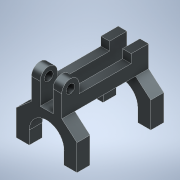
# Autodesk Inventor part: TransferFork
Saved by Autodesk Inventor 2022.2 (Build 262287030, 287C)
## iProperties
Created: 2023-03-20
Part Number: TransferFork
Material: Iron, Cast
Document SubType Name: Modeling
Designer: jak27277
Density: 7.15 g/cm^3
Appearance: Iron Gray
Author: jak27277
Autodesk Inventor part; units mm, degrees
ref_plane "YZ Plane" through (0, 0, 0) normal (1, 0, 0) x (0, 1, 0)
ref_plane "XZ Plane" through (0, 0, 0) normal (0, 1, 0) x (-1, 0, 0)
ref_plane "XY Plane" through (0, 0, 0) normal (0, 0, 1) x (1, 0, 0)
sketch "Sketch1" plane through (0, 0, 0) normal (0, 0, 1) x (1, 0, 0)
  arc A0 (25.4, 0) -> (-25.4, 0) centre (0, 0) ccw
  line L0 (-25.4, 0) -> (-25.4, -19.05)
  line L1 (-25.4, -19.05) -> (-44.45, -19.05)
  line L2 (-44.45, -19.05) -> (-44.45, 19.05)
  line L3 (-44.45, 19.05) -> (-22.225, 38.1)
  line L4 (-22.225, 38.1) -> (-22.225, 69.85)
  line L5 (-22.225, 69.85) -> (-9.525, 69.85)
  line L6 (-9.525, 69.85) -> (-9.525, 38.1)
  line L7 (-9.525, 38.1) -> (0, 38.1)
  line L8 (0, 38.1) -> (0, -30.0357)
  line L9 (25.4, 0) -> (25.4, -19.05)
  line L10 (25.4, -19.05) -> (44.45, -19.05)
  line L11 (44.45, -19.05) -> (44.45, 19.05)
  line L12 (44.45, 19.05) -> (22.225, 38.1)
  line L13 (22.225, 38.1) -> (22.225, 69.85)
  line L14 (9.525, 69.85) -> (9.525, 38.1)
  line L15 (22.225, 69.85) -> (9.525, 69.85)
  line L16 (9.525, 38.1) -> (0, 38.1)
  dimension "d0" = 88.9
  dimension "d1" = 19.05
  dimension "d2" = 38.1
  dimension "d3" = 31.75
  dimension "d4" = 19.05
  dimension "d5" = 25.4
  dimension "d6" = 88.9
  dimension "d7" = 19.05
  dimension "d8" = 44.45
  constraints: 34 end point, 7 symmetric about line, 6 perpendicular, 2 parallel, 2 point on circle, 2 tangent, 2 vertical, 1 centre point, 1 coincident
  measures "d0" distance between parallel lines of L11 L2
  measures "d1" distance of L0.start L0.end
  measures "d2" distance of L11.start L11.end
  measures "d3" distance of L13.start L13.end
  measures "d4" distance of L0.end L1.end
  measures "d5" radius of A0
  measures "d6" distance between parallel lines of L10 L15
  measures "d7" distance between parallel lines of L14 L6
  measures "d8" distance between parallel lines of L13 L4
extrude "Extrusion1" add sketch "Sketch1" against normal blind 127
sketch "Sketch3" plane through (44.45, -19.05, 0) normal (1, 0, 0) x (0, 0, -1)
  line L0 (0, 88.9) -> (127, 88.9) projected
  line L1 (25.4, 88.9) -> (101.6, 88.9)
  line L2 (101.6, 88.9) -> (101.6, 76.2)
  line L3 (101.6, 76.2) -> (25.4, 76.2)
  line L4 (25.4, 76.2) -> (25.4, 88.9)
  line L5 (127, 88.9) -> (127, 57.15) projected
  line L6 (0, 57.15) -> (0, 88.9) projected
  line L7 (0, 0) -> (127, 0) projected
  line L8 (0, 57.15) -> (127, 57.15) projected
  line L9 (19.05, 0) -> (107.95, 0)
  line L10 (107.95, 0) -> (107.95, 57.15)
  line L11 (107.95, 57.15) -> (19.05, 57.15)
  line L12 (19.05, 57.15) -> (19.05, 0)
  line L13 (127, 38.1) -> (127, 0) projected
  line L14 (0, 0) -> (0, 38.1) projected
  point P0 (0, 19.05)
  point P1 (101.6, 82.55)
  point P2 (107.95, 0)
  dimension "d12" = 25.4
  dimension "d13" = 25.4
  dimension "d14" = 12.7
  dimension "d15" = 19.05
  dimension "d16" = 19.05
  constraints: 16 end point, 4 parallel, 3 point on line, 2 horizontal, 2 perpendicular, 1 midpoint
  measures "d12" distance from line of point (101.6, 82.55) L5
  measures "d13" distance between parallel lines of L4 L6
  measures "d14" distance of L1.end L2.end
  measures "d15" distance between parallel lines of L10 L13
  measures "d16" distance between parallel lines of L14 L12
extrude "Extrusion2" cut sketch "Sketch3" against normal through all contours L0 L2 L3 L4 | L8 L10 L7 L12
sketch "Sketch4" plane through (22.225, 38.1, 0) normal (1, 0, 0) x (0, 0, -1)
  line L0 (0, 31.75) -> (25.4, 31.75) projected
  arc A0 (25.4, 31.75) -> (0, 31.75) centre (12.7, 31.75) ccw
  point P0 (0, -38.1)
  constraints: 2 point on circle, 1 centre point, 1 midpoint
extrude "Extrusion3" add sketch "Sketch4" against normal up to surface (12.7 mm away)
mirror "Mirror1" about plane through (0, 0, 0) normal (1, 0, 0) of "Extrusion3"
sketch "Sketch5" plane through (22.225, 38.1, -127) normal (1, 0, 0) x (0, 0, -1)
  arc A0 (-101.6, 31.75) -> (-127, 31.75) centre (-114.3, 31.75) ccw projected
  point P0 (-127, -38.1)
  constraints: 1 coincident
hole "Hole1" at (22.225, 69.85, -12.7) direction (-1, 0, 0) diameter 12.7 end through all
body "Solid1"
